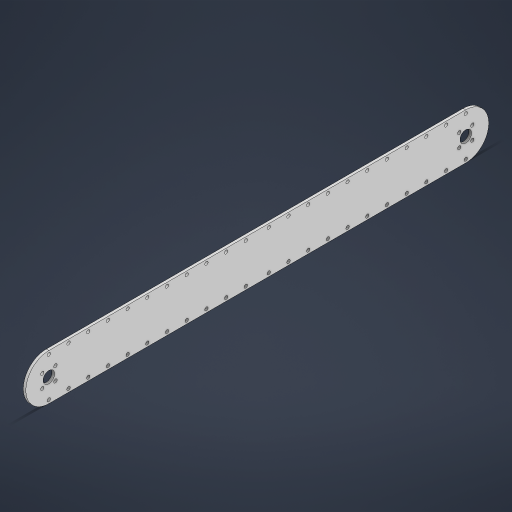
# Autodesk Inventor part: SecondStageArmBar1
Saved by Autodesk Inventor 2024 (Build 280153000, 153)
## iProperties
Created: 2024-01-27
Part Number: SecondStageArmBar1
Material: Generic
Document SubType Name: Modeling
Designer: avsar
Density: 1 g/cm^3
Appearance: Default
Author: avsar
Autodesk Inventor part; units mm, degrees
ref_plane "YZ Plane" through (0, 0, 0) normal (1, 0, 0) x (0, 1, 0)
ref_plane "XZ Plane" through (0, 0, 0) normal (0, 1, 0) x (-1, 0, 0)
ref_plane "XY Plane" through (0, 0, 0) normal (0, 0, 1) x (1, 0, 0)
sketch "Sketch1" plane through (0, 0, 0) normal (1, 0, 0) x (0, 1, 0)
  line L0 (-28, 254) -> (28, 254) construction
  line L1 (28, 254) -> (28, -254)
  line L2 (28, -254) -> (-28, -254) construction
  line L3 (-28, -254) -> (-28, 254)
  line L4 (-28, 254) -> (28, -254) construction
  line L5 (28, 254) -> (-28, -254) construction
  arc A0 (28, 254) -> (-28, 254) centre (0, 254) ccw
  arc A1 (-28, -254) -> (28, -254) centre (0, -254) ccw
  circle A2 centre (0, 254) radius 7
  circle A3 centre (8, 262) radius 2.05
  circle A4 centre (-8, 262) radius 2.05
  circle A5 centre (-8, 246) radius 2.05
  circle A6 centre (8, 246) radius 2.05
  circle A7 centre (0, -254) radius 7
  circle A8 centre (8, -246) radius 2.05
  circle A9 centre (-8, -246) radius 2.05
  circle A10 centre (-8, -262) radius 2.05
  circle A11 centre (8, -262) radius 2.05
  point P0 (0, 0)
  dimension "d0" = 56
  dimension "d1" = 508
  dimension "d2" = 14
  dimension "d3" = 4.1
  dimension "d4" = 8
  dimension "d5" = 8
  dimension "d8" = 360
  dimension "d10" = 14
  dimension "d11" = 4.1
  dimension "d12" = 8
  dimension "d13" = 8
  dimension "d16" = 360
  constraints: 12 centre point, 12 end point, 4 midpoint, 4 point on circle, 4 tangent, 2 coincident, 2 parallel, 1 horizontal, 1 perpendicular, 18 other
  measures "d0" distance of L1.end L2.end
  measures "d1" distance of L0.end L1.end
  measures "d2" diameter of A2
  measures "d3" diameter of A3
  measures "d4" horizontal distance of point (0, 254) A3.centre
  measures "d5" horizontal distance of A0.centre A3.centre
  measures "d10" diameter of A7
  measures "d11" diameter of A8
  measures "d12" horizontal distance of A8.centre point (0, -254)
  measures "d13" horizontal distance of point (0, -254) A8.centre
extrude "Extrusion1" add sketch "Sketch1" along normal blind 3.175
sketch "Sketch2" plane through (3.175, 0, 0) normal (1, 0, 0) x (0, 0, -1)
  circle A0 centre (-254, 24) radius 2
  circle A1 centre (-254, 0) radius 7 construction
  line L0 (254, 28) -> (-254, 28) construction
  circle A2 centre (-230, 24) radius 2
  circle A3 centre (-206, 24) radius 2
  circle A4 centre (-182, 24) radius 2
  circle A5 centre (-158, 24) radius 2
  circle A6 centre (-134, 24) radius 2
  circle A7 centre (-110, 24) radius 2
  circle A8 centre (-86, 24) radius 2
  circle A9 centre (-62, 24) radius 2
  circle A10 centre (-38, 24) radius 2
  circle A11 centre (-14, 24) radius 2
  line L1 (0, 28) -> (0, -28) construction
  line L2 (-254, -28) -> (254, -28) construction
  arc A12 (-254, 28) -> (-254, -28) centre (-254, 0) ccw construction
  circle A13 centre (254, 0) radius 7 construction
  line L3 (-254, 0) -> (254, 0) construction
  circle A14 centre (254, 24) radius 2
  circle A15 centre (230, 24) radius 2
  circle A16 centre (206, 24) radius 2
  circle A17 centre (182, 24) radius 2
  circle A18 centre (158, 24) radius 2
  circle A19 centre (134, 24) radius 2
  circle A20 centre (110, 24) radius 2
  circle A21 centre (86, 24) radius 2
  circle A22 centre (62, 24) radius 2
  circle A23 centre (38, 24) radius 2
  circle A24 centre (14, 24) radius 2
  circle A25 centre (-254, -24) radius 2
  circle A26 centre (-230, -24) radius 2
  circle A27 centre (-206, -24) radius 2
  circle A28 centre (-182, -24) radius 2
  circle A29 centre (-158, -24) radius 2
  circle A30 centre (-134, -24) radius 2
  circle A31 centre (-110, -24) radius 2
  circle A32 centre (-86, -24) radius 2
  circle A33 centre (-62, -24) radius 2
  circle A34 centre (-38, -24) radius 2
  circle A35 centre (-14, -24) radius 2
  circle A36 centre (254, -24) radius 2
  circle A37 centre (230, -24) radius 2
  circle A38 centre (206, -24) radius 2
  circle A39 centre (182, -24) radius 2
  circle A40 centre (158, -24) radius 2
  circle A41 centre (134, -24) radius 2
  circle A42 centre (86, -24) radius 2
  circle A43 centre (62, -24) radius 2
  circle A44 centre (38, -24) radius 2
  circle A45 centre (14, -24) radius 2
  circle A46 centre (110, -24) radius 2
  point P0 (0, 0)
  dimension "d20" = 4
  dimension "d21" = 4
  dimension "d24" = 24
  constraints: 44 centre point, 33 symmetric about line, 4 end point, 2 horizontal, 2 midpoint, 1 vertical alignment, 53 other
  measures "d20" diameter of A0
  measures "d21" distance from line of L0 A0.centre
  measures "d24" distance of A0.centre A2.centre
extrude "Extrusion2" cut sketch "Sketch2" against normal through all
body "Solid1"
